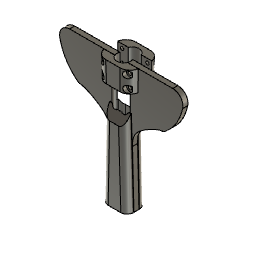
Pinpong handle with shaft connector (Autodesk Fusion 360 design; units mm, degrees)
Autodesk Fusion 360 part; units mm, degrees
note: some values were not read from the file. Chosen so that the rebuilt part matches the saved one: which bodies a step acts on; which face or edge a step refers to. Set by a fixed rule: which sketch regions a step uses.
sketch "Sketch2" plane through (0, 0, 0) normal (0, 1, 0) x (1, 0, 0)
  line L0 (12.5, -100) -> (-12.5, -100)
  line L1 (14.5, 0) -> (-15.5, 0)
  line L2 (12.5, -100) -> (14.5, 0)
  line L3 (-12.5, -100) -> (-15.5, 0)
  dimension "d8" = 25
  dimension "d20" = 30
  constraint horizontal L0
  constraint horizontal L1
  measures "d8" distance of L0.start L0.end
  measures "d20" distance of L1.start L1.end
extrude "Extrude2" add sketch "Sketch2" along normal blind 16 makes body 1
fillet "Fillet1" radius 7.5 1 edges at (13.5, 16, 50) on bodies 1
fillet "Fillet1" radius 7.5 3 edges at (-14, 16, 50) (13.5, 0, 50) (-14, 0, 50) on bodies 1
ref_plane "WorkPlane2" through (0, 8, 0) normal (0, 1, 0) x (0, 0, 1)
split "Split2" by plane through (0, 8, 0) normal (0, 1, 0) bodies 1 makes body 2 at (-1.9983, 16, 33.3333)
move_body "Move11" bodies 2 to x (1, 0, 0) y (0, 0.866025, -0.5) z (0, 0.5, 0.866025) at (0, -49.55, -23.6795)
split "Split3" by plane through (0, 8, 0) normal (0, 1, 0) bodies 2 makes body 3 at (-1.6655, 10.1021, 57.3504)
move_body "Move12" bodies 2 to x (1, 0, 0) y (0, 0.866025, 0.5) z (0, -0.5, 0.866025) at (0.5, -16.8068, 24.3342)
delete_body "RemoveBody1" bodies 3
delete_body "RemoveBody2" bodies 1
copy_body "CopyPasteBodies1" bodies 2 makes body 4
move_body "Move13" bodies 4 to x (-1, 0, 0) y (0, -1, 0) z (0, 0, 1) at (0, -131.2436, 0)
sketch "Sketch3" plane through (0, 0, 0) normal (0, 1, 0) x (1, 0, 0)
  line L0 (100, -100) -> (75, -100)
  line L1 (102.5, 0) -> (72.5, 0)
  line L2 (100, -100) -> (102.5, 0)
  line L3 (75, -100) -> (72.5, 0)
  line L4 (162.5, -150) -> (12.5, -150)
  line L5 (137.5, -100) -> (37.5, -100)
  spline S0 degree 5 poles (162.5, -150) (162.3299, -147.956) (161.8933, -143.8732) (160.9491, -137.7644) (159.0712, -129.652) (155.1878, -119.5928) (150.0779, -111.6516) (144.5527, -105.7854) (139.9965, -101.9207) (137.5, -100) knots 0 0 0 0 0 0 0.2 0.4 0.6 0.8 1 1 1 1 1 1
  line L6 (144.3115, -105.2406) -> (130.6885, -94.7594)
  spline S1 degree 5 poles (137.5, -100) (137.095, -100.0831) (136.1629, -100.1512) (134.3978, -99.9592) (131.3042, -99.1073) (126.2081, -97.0136) (120.1473, -93.9368) (113.5863, -89.9927) (107.895, -85.6593) (103.9841, -81.2752) (101.7549, -76.8007) (101.0113, -73.0287) (100.8112, -70.0004) (100.803, -67.8791) (100.8302, -66.7927) knots 0 0 0 0 0 0 0.1 0.2 0.3 0.4 0.5 0.6 0.7 0.8 0.9 1 1 1 1 1 1
  line L7 (120.1856, -94.1551) -> (108.5156, -86.3751)
  line L8 (100.7077, -71.6928) -> (100.9527, -61.8926)
  spline S2 degree 5 poles (12.5, -150) (12.6701, -147.956) (13.1067, -143.8732) (14.0509, -137.7644) (15.9288, -129.652) (19.8122, -119.5928) (24.9221, -111.6516) (30.4473, -105.7854) (35.0035, -101.9207) (37.5, -100) knots 0 0 0 0 0 0 0.2 0.4 0.6 0.8 1 1 1 1 1 1
  line L9 (162.9704, -155.6537) -> (162.0296, -144.3463)
  line L10 (12.0296, -155.6537) -> (12.9704, -144.3463)
  line L11 (30.6885, -105.2406) -> (44.3115, -94.7594)
  spline S3 degree 5 poles (37.5, -100) (37.905, -100.0831) (38.8371, -100.1512) (40.6022, -99.9592) (43.6958, -99.1073) (48.7919, -97.0136) (54.8527, -93.9368) (61.4137, -89.9927) (67.105, -85.6593) (71.0159, -81.2752) (73.2451, -76.8007) (73.9887, -73.0287) (74.1888, -70.0004) (74.197, -67.8791) (74.1698, -66.7927) knots 0 0 0 0 0 0 0.1 0.2 0.3 0.4 0.5 0.6 0.7 0.8 0.9 1 1 1 1 1 1
  line L12 (139.3752, -99.6154) -> (135.6248, -100.3846)
  line L13 (35.6248, -99.6154) -> (39.3752, -100.3846)
  line L14 (54.8144, -94.1551) -> (66.4844, -86.3751)
  line L15 (74.2923, -71.6928) -> (74.0473, -61.8926)
  point P0 (114.3506, -90.2651)
  point P1 (60.6494, -90.2651)
  dimension "d16" = 25
  constraint horizontal L0
  constraint horizontal L1
  constraint horizontal L4
  constraint parallel L0 L5
  constraint midpoint L5.start L6
  constraint coincident L2 S1.end
  constraint midpoint P0 L7
  constraint midpoint S1.end L8
  constraint coincident L2 L8.end
  constraint midpoint L4.start L9
  constraint midpoint L5.start L12
  measures "d16" distance of L0.start L0.end
extrude "Extrude3" add sketch "Sketch3" along normal blind 6 separate body contours L0 L4 L5 S0 S1 S2 S3 | L0 L1 L2 L3 L5 L8 L15 | L2 L5 S1 L8 | L3 L5 S3 L15 makes body 5
move_body "Move14" bodies 2 4 to x (1, 0, 0) y (0, 1, 0) z (0, 0, 1) at (87.5, 70, -4.5)
move_body "Align1" bodies 4 to x (1, 0, 0) y (0, 1, 0) z (0, 0, 1) at (0, 21.365, 25.4479)
move_body "Align2" bodies 2 to x (1, 0, 0) y (0, 1, 0) z (0, 0, 1) at (0, -24.1214, 25.4479)
combine "Combine3" operation add target body 2 tool bodies 4 5
move_body "Align7" bodies 2 to x (1, 0, 0) y (0, 1, 0) z (0, 0, 1) at (-87.5, -3, 0)
ref_plane "WorkPlane5" through (0, 3, 75) normal (0, -1, 0) x (-1, 0, 0)
sketch "Sketch8" plane through (0, 0, 0) normal (0, 0, -1) x (1, 0, 0)
  line L0 (-15, -3) -> (-15, -3.5)
  ellipse E0 centre (-7.4966, -3.5) end of major axis (-15, -3.5) minor radius 7.5 (-15, -3.5) -> (-7.4966, -11) ccw
  line L1 (-7.4966, -11) -> (7.4985, -11)
  ellipse E1 centre (7.4985, -3.5) end of major axis (15, -3.5) minor radius 7.5 (7.4985, -11) -> (15, -3.5) ccw
  line L2 (15, -3.5) -> (15, -3)
  line L3 (15, -3) -> (15, 3)
  line L4 (15, 3) -> (15, 3.5)
  ellipse E2 centre (7.4966, 3.5) end of major axis (15, 3.5) minor radius 7.5 (15, 3.5) -> (7.4966, 11) ccw
  line L5 (7.4966, 11) -> (-7.4985, 11)
  ellipse E3 centre (-7.4985, 3.5) end of major axis (-15, 3.5) minor radius 7.5 (-7.4985, 11) -> (-15, 3.5) ccw
  line L6 (-15, 3.5) -> (-15, 3)
  line L7 (-15, 3) -> (-15, -3)
  circle A0 centre (-5.5, 0) radius 5.5
  circle A1 centre (5.5, 0) radius 5.5
  line L8 (-5.5, 5) -> (5.5, 5)
  line L9 (-5.5, -5) -> (5.5, -5)
  circle A2 centre (-9, 0) radius 3.5
  circle A3 centre (9, 0) radius 3.5
  dimension "d46" = 11
  dimension "d47" = 11
  dimension "d93" = 11
  dimension "d106" = 7
  dimension "d107" = 7
  constraint horizontal L8
  constraint horizontal L9
  measures "d46" diameter of A0
  measures "d47" diameter of A1
  measures "d93" distance of L8.start L8.end
  measures "d106" diameter of A2
  measures "d107" diameter of A3
sketch "Sketch10" plane through (0, 0, 0) normal (0, 0, 1) x (1, 0, 0)
  line L0 (120, 20) -> (160, 20)
  line L1 (160, 20) -> (160, -5)
  line L2 (160, -5) -> (120, -5)
  line L3 (120, -5) -> (120, 20)
  dimension "d57" = 25
  dimension "d58" = 40
  constraint horizontal L0
  constraint vertical L1
  constraint horizontal L2
  constraint vertical L3
  measures "d57" distance of L0.start L2.end
  measures "d58" distance of L0.start L0.end
extrude "Extrude7" add sketch "Sketch10" along normal blind 25 draft 1 separate body makes body 6
move_body "Align8" bodies 6 to x (1, 0, 0) y (0, 1, 0) z (0, 0, 1) at (-140, -7.5, -12.6164)
move_body "Move20" bodies 6 to x (1, 0, 0) y (0, 1, 0) z (0, 0, 1) at (0, 0, 137.5)
extrude "Extrude8" cut sketch "Sketch8" against normal blind 125 contours A0 A2 | A0 A2 | A1 A3 | A1 A3 picked at (-9.1566, 0) picked at (-11.4899, 0) picked at (11.4709, -0.4161) picked at (9.1777, -0.4949) bodies 2
ref_plane "WorkPlane8" through (0, 0, 35) normal (0, 0, 1) x (1, 0, 0)
sketch "Sketch14" plane through (0, 0, 35) normal (0, 0, 1) x (1, 0, 0)
  circle A0 centre (-5.5, 0) radius 5.5
  circle A1 centre (5.5, 0) radius 5.5
  line L0 (-5.5, -5) -> (5.5, -5)
  line L1 (-5.5, 5) -> (5.5, 5)
  line L2 (-4, -2) -> (4, -2)
  line L3 (4, -2) -> (4, -5)
  line L4 (4, -5) -> (-4, -5)
  line L5 (-4, -5) -> (-4, -2)
  dimension "d98" = 11
  dimension "d99" = 11
  dimension "d100" = 11
  dimension "d103" = 3
  constraint horizontal L0
  constraint horizontal L1
  constraint horizontal L2
  constraint vertical L3
  constraint horizontal L4
  constraint vertical L5
  measures "d98" diameter of A0
  measures "d99" diameter of A1
  measures "d100" distance of L1.start L1.end
  measures "d103" distance of L2.start L4.end
extrude "Extrude13" cut sketch "Sketch14" along normal blind 90 bodies 2
extrude "Extrude14" cut sketch "Sketch14" against normal blind 35 contours A0 A1 L0 L2 L4 | A0 L0 L2 L4 L5 | A1 L0 L2 L3 L4 picked at (-3.5295, -3.8887) picked at (3.5295, -3.8887) bodies 2
sketch "Sketch11" plane through (0, 0, 149.8836) normal (0, 0, 1) x (-1, 0, 0)
  line L0 (20.4364, -12.9364) -> (20.4364, 12.9364)
  line L1 (20.4364, 12.9364) -> (-20.4364, 12.9364)
  line L2 (-20.4364, 12.9364) -> (-20.4364, -12.9364)
  line L3 (-20.4364, -12.9364) -> (20.4364, -12.9364)
  circle A0 centre (0, 0) radius 8.15
  dimension "d60" = 16.3
  constraint coincident A0.centre origin
  measures "d60" diameter of A0
extrude "Extrude9" cut sketch "Sketch11" along normal blind -45 and the other way blind -5 contours A0 bodies 2 6
sketch "Sketch12" plane through (0, -10.317, -0.1801) normal (0, -0.999848, -0.017452) x (1, 0, 0)
  line L0 (20.4364, 150.0865) -> (-20.4364, 150.0865)
  line L1 (-20.4364, 150.0865) -> (-20, 125.0827)
  line L2 (-20, 125.0827) -> (20, 125.0827)
  line L3 (20, 125.0827) -> (20.4364, 150.0865)
  circle A0 centre (-15, 145) radius 2
  circle A1 centre (-15, 130) radius 2
  circle A2 centre (15, 145) radius 2
  circle A3 centre (15, 130) radius 2
  circle A4 centre (-15, 145) radius 4
  circle A5 centre (-15, 130) radius 4
  circle A6 centre (15, 130) radius 4
  circle A7 centre (15, 145) radius 4
  dimension "d65" = 4
  dimension "d66" = 4
  dimension "d67" = 4
  dimension "d68" = 4
  dimension "d69" = 8
  dimension "d70" = 8
  dimension "d71" = 8
  dimension "d72" = 8
  constraint concentric A0 A4
  measures "d65" diameter of A0
  measures "d66" diameter of A1
  measures "d67" diameter of A2
  measures "d68" diameter of A3
  measures "d69" diameter of A4
  measures "d70" diameter of A5
  measures "d71" diameter of A7
  measures "d72" diameter of A6
extrude "Extrude10" cut sketch "Sketch12" against normal blind 30 contours A0 | A1 | A2 | A3 bodies 2 6
extrude "Extrude11" cut sketch "Sketch12" against normal blind 5 contours A4 | A5 | A6 | A7 bodies 6
sketch "Sketch13" plane through (0, 10.317, -0.1801) normal (0, 0.999848, -0.017452) x (-1, 0, 0)
  ellipse E0 centre (15, 130.4396) end of major axis (15, 128.4384) minor radius 2
  ellipse E1 centre (-15, 145.4487) end of major axis (-15, 143.4475) minor radius 2
  ellipse E2 centre (15, 145.4487) end of major axis (15, 143.4475) minor radius 2
  ellipse E3 centre (-15, 130.4396) end of major axis (-15, 128.4384) minor radius 2
  line L0 (20.4364, 150.0865) -> (-20.4364, 150.0865)
  line L1 (-20.4364, 150.0865) -> (-20, 125.0827)
  line L2 (-20, 125.0827) -> (20, 125.0827)
  line L3 (20, 125.0827) -> (20.4364, 150.0865)
  circle A0 centre (-15, 145) radius 4
  circle A1 centre (15, 145) radius 4
  circle A2 centre (15, 130) radius 4
  circle A3 centre (-15, 130) radius 4
  dimension "d83" = 8
  dimension "d87" = 8
  dimension "d88" = 8
  dimension "d89" = 8
  measures "d83" diameter of A0
  measures "d87" diameter of A1
  measures "d88" diameter of A3
  measures "d89" diameter of A2
extrude "Extrude12" cut sketch "Sketch13" against normal blind 5 contours E0 | E1 | E2 | E3 | A0 | A1 | A2 | A3 bodies 6
fillet "Fillet3" radius 12 2 edges at (75, 0, 150) (-75, 0, 150) on bodies 2 6
fillet "Fillet3" radius 12 4 edges at (20.2182, 12.7182, 137.3836) (-20.2182, 12.7182, 137.3836) (20.2182, -12.7182, 137.3836) (-20.2182, -12.7182, 137.3836) on bodies 2 6
combine "Combine4" operation add target body 6 tool bodies 2
split "Split4" by plane through (0, 3, 75) normal (0, -1, 0) bodies 6 makes body 7 at (5.2279, 6.2523, 133.2169) makes body 8 at (-49.1279, 3, 133.2263)
ref_plane "WorkPlane6" through (0, -3, 75) normal (0, -1, 0) x (-1, 0, 0)
split "Split5" by plane through (0, -3, 75) normal (0, -1, 0) bodies 8 makes body 9 at (49.1714, -3, 135.3079) makes body 10 at (7.2423, -3.7378, 141.5502) makes body 11 at (1.6244, -11, 29.1291) makes body 12 at (2.3991, 3, 23.3333)
move_body "Move21" bodies 7 to x (1, 0, 0) y (0, 1, 0) z (0, 0, 1) at (0, 10, 0)
combine "Combine5" operation add target body 6 tool bodies 8 11 9 12 10
